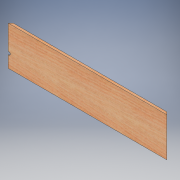
# Autodesk Inventor part: SkinnySideWidthOutlet
Saved by Autodesk Inventor 2016 (Build 200138000, 138)
## iProperties
Created: 2016-02-11
Part Number: SkinnySideWidthOutlet
Material: Wood (Birch)
Document SubType Name: Modeling
Designer: ron
Density: 0.55 g/cm^3
Appearance: Birch - Natural Polished
Mass: 862.606 g
Surface Area: 2217.66 cm^2
Volume: 1568.37 cm^3
Author: ron
Autodesk Inventor part; units mm, degrees
ref_plane "YZ Plane" through (0, 0, 0) normal (1, 0, 0) x (0, 1, 0)
ref_plane "XZ Plane" through (0, 0, 0) normal (0, 1, 0) x (-1, 0, 0)
sketch "Sketch1" plane through (0, 0, 0) normal (1, 0, 0) x (0, 1, 0)
  line L0 (0, 0) -> (155.1, 0)
  line L1 (155.1, 0) -> (155.1, -10)
  line L2 (0, -20) -> (0, 0)
  line L3 (155.1, -10) -> (101.6, -10)
  line L4 (101.6, -10) -> (101.6, -20)
  line L5 (101.6, -20) -> (0, -20)
  dimension "d0" = 53.5
  dimension "d1" = 155.1
  dimension "d2" = 10
  dimension "d3" = 10
  dimension "d4" = 20
  constraints: 12 end point, 3 horizontal, 2 parallel, 1 perpendicular
  measures "d0" distance of L1.end L3.end
  measures "d1" distance between parallel lines of L1 L2
  measures "d2" distance between parallel lines of L3 L5
  measures "d3" distance between parallel lines of L0 L3
  measures "d4" vertical distance of L4.end L0.end
extrude "Extrusion1" add sketch "Sketch1" along normal blind 629.2342
chamfer "Chamfer1" distance 19.812 angle 45 1 edges at (629.2342, 50.8, -20)
chamfer "Chamfer2" distance 19.812 angle 45 1 edges at (0, 50.8, -20)
ref_plane "Work Plane4" through (55.733, 38.0112, -55.921) normal (0.7071, 0, -0.7071) x (0, -1, 0)
sketch "Sketch3" plane through (55.733, 38.0112, -55.921) normal (0.7071, 0, -0.7071) x (0, -1, 0)
  line L0 (-63.5888, 0) -> (-63.5888, -416.9174) projected
  line L1 (-63.5888, 0) -> (38.0112, 0) projected
  line L2 (-117.0888, -0.1329) -> (-117.0888, -445.0687) projected
  line L3 (-117.0888, -0.1329) -> (-14.7014, -0.1329)
  line L4 (38.0112, -0.1329) -> (-117.0888, -0.1329) projected
  dimension "d18" = 102.3874
  constraints: 2 end point, 1 point on line
  measures "d18" distance of L2.start L3.end
hole "Hole1" at (55.827, 52.7126, -55.827) direction (-0.7071, 0, 0.7071) diameter 12.7 depth 127 tip angle 118
body "Solid1"
